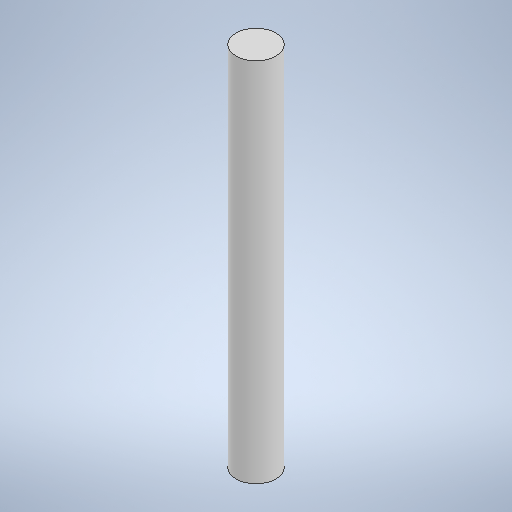
# Autodesk Inventor part: 0.5 and 4 inch stand
Saved by Autodesk Inventor 2025.2 (Build 292293000, 293)
## iProperties
Created: 2024-11-22
Part Number: 0.5 and 4 inch stand
Material: Generic
Document SubType Name: Modeling
Designer: dgpark2
Density: 1 g/cm^3
Appearance: Default
Author: dgpark2
Autodesk Inventor part; units mm, degrees
ref_plane "YZ Plane" through (0, 0, 0) normal (1, 0, 0) x (0, 1, 0)
ref_plane "XZ Plane" through (0, 0, 0) normal (0, 1, 0) x (-1, 0, 0)
ref_plane "XY Plane" through (0, 0, 0) normal (0, 0, 1) x (1, 0, 0)
sketch "Sketch1" plane through (0, 0, 0) normal (0, 1, 0) x (-1, 0, 0)
  circle A0 centre (10.616, 8.5359) radius 6.2865
  circle A1 centre (-1.2752, 0.6307) radius 0.5481
  circle A2 centre (0, 13.4135) radius 0.0717
  point P0 (0, 0)
  dimension "d1" = 12.573
  constraints: 3 centre point
  measures "d1" diameter of A0
extrude "Extrusion1" add sketch "Sketch1" along normal blind 115 contours A0
body "Solid1"
